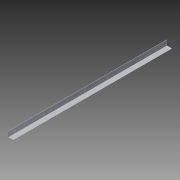
# Autodesk Inventor part: Electrical Board 1 Bracing L Channel
Saved by Autodesk Inventor 2014 SP1 (Build 180222100, 222)
## iProperties
Created: 2013-10-26
Part Number: Electrical Board 1 Bracing L Channel
Material: Aluminum 6061
Document SubType Name: Modeling
Designer: Moses
Density: 2.71 g/cm^3
Appearance: Aluminum - Flat
Mass: 31.3445 g
Surface Area: 300.339 cm^2
Volume: 11.5662 cm^3
Author: Moses
Autodesk Inventor part; units mm, degrees
ref_plane "YZ Plane" through (0, 0, 0) normal (1, 0, 0) x (0, 1, 0)
ref_plane "XZ Plane" through (0, 0, 0) normal (0, 1, 0) x (-1, 0, 0)
ref_plane "XY Plane" through (0, 0, 0) normal (0, 0, 1) x (1, 0, 0)
sketch "Sketch1" plane through (0, 0, 0) normal (0, 0, 1) x (1, 0, 0)
  line L0 (0, 0) -> (15.875, 0)
  line L1 (15.875, 0) -> (15.875, 0.7937)
  line L2 (15.875, 0.7937) -> (0.7938, 0.7937)
  line L3 (0.7938, 0.7937) -> (0.7937, 15.875)
  line L4 (0.7937, 15.875) -> (0, 15.875)
  line L5 (0, 15.875) -> (0, 0)
  dimension "d0" = 15.875
  dimension "d1" = 0.7937
  dimension "d2" = 0.7937
  constraints: 12 end point, 4 perpendicular, 2 parallel, 1 horizontal
  measures "d0" distance of L0.start L0.end
  measures "d1" distance of L0.end L1.end
  measures "d2" distance of L3.end L4.end
extrude "Extrusion1" add sketch "Sketch1" along normal blind 474.6752
sketch "Sketch2" plane through (0.7937, 0.7937, 0) normal (1, 0, 0) x (0, 0, -1)
  line L0 (0, 0) -> (0, 15.0812) projected
  line L1 (-474.6752, 0) -> (-474.6752, 15.0812) projected
  circle A0 centre (-19.0627, 7.5406) radius 2.2479 projected
  circle A1 centre (-63.5127, 7.5406) radius 2.2479 projected
  line L2 (0, 7.5406) -> (-474.6752, 7.5406) construction
  circle A2 centre (-6.35, 7.5406) radius 2.2479
  circle A3 centre (-82.55, 7.5406) radius 2.2479
  circle A4 centre (-246.0752, 7.5406) radius 2.2479
  circle A5 centre (-455.6252, 7.5406) radius 2.2479
  circle A6 centre (-347.6752, 7.5406) radius 2.2479
  circle A7 centre (-369.6843, 8.0867) radius 1.905 projected
  point P0 (0, -0.7937)
  dimension "d5" = 4.4958
  dimension "d8" = 19.05
  dimension "d9" = 127
  dimension "d10" = 228.6
  dimension "d11" = 6.35
  dimension "d12" = 82.55
  constraints: 5 centre point, 5 equal radius, 5 point on line, 2 end point, 2 midpoint
  measures "d5" diameter of A0
  measures "d8" distance from line of A5.centre L1
  measures "d9" distance of A6.centre L2.end
  measures "d10" distance of L2.end A4.centre
  measures "d11" distance from line of L0 A2.centre
  measures "d12" distance from line of L0 A3.centre
extrude "Extrusion2" cut sketch "Sketch2" against normal through all
body "Solid1"
